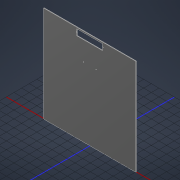
# Autodesk Inventor part: Panel Back
Saved by Autodesk Inventor 2022.2 (Build 262287010, 287A)
## iProperties
Created: 2022-03-16
Part Number: Panel Back
Material: Polycarbonat, klar
Document SubType Name: Modeling
Designer: sleib
Density: 1.2 g/cm^3
Appearance: Glatt - Schwarz
Author: sleib
Autodesk Inventor part; units mm, degrees
ref_plane "YZ Plane" through (0, 0, 0) normal (1, 0, 0) x (0, 1, 0)
ref_plane "XZ Plane" through (0, 0, 0) normal (0, 1, 0) x (-1, 0, 0)
ref_plane "XY Plane" through (0, 0, 0) normal (0, 0, 1) x (1, 0, 0)
sketch "Skizze1" plane through (0, 0, 0) normal (0, 0, 1) x (1, 0, 0)
  line L0 (-242, -252) -> (242, -252)
  line L1 (242, -252) -> (242, 252)
  line L2 (242, 252) -> (-242, 252)
  line L3 (-242, 252) -> (-242, -252)
  line L4 (-242, -252) -> (242, 252) construction
  line L5 (242, -252) -> (-242, 252) construction
  line L6 (-67.5, 245) -> (67.5, 245)
  line L7 (67.5, 213) -> (-67.5, 213)
  line L8 (0, 245) -> (0, 213) construction
  line L9 (69.1, 229) -> (-69.1, 229) construction
  line L10 (-69.1, 230.7) -> (-67.5, 230.7)
  line L11 (-69.1, 227.3) -> (-67.5, 227.3)
  line L12 (69.1, 230.7) -> (67.5, 230.7)
  line L13 (69.1, 227.3) -> (67.5, 227.3)
  line L14 (67.5, 245) -> (67.5, 230.7)
  line L15 (67.5, 227.3) -> (67.5, 213)
  arc A0 (69.1, 227.3) -> (69.1, 230.7) centre (69.1, 229) ccw
  arc A1 (-69.1, 230.7) -> (-69.1, 227.3) centre (-69.1, 229) ccw
  line L16 (-67.5, 230.7) -> (-67.5, 245)
  line L17 (-67.5, 213) -> (-67.5, 227.3)
  circle A2 centre (-33.4649, 111.0916) radius 1.7
  circle A3 centre (33.465, 111.0916) radius 1.7
  point P0 (0, 0)
  point P1 (0, 252)
  point P2 (0, 229)
  dimension "d0" = 484
  dimension "d1" = 504
  dimension "d6" = 135
  dimension "d7" = 32
  dimension "d8" = 138.2
  dimension "d10" = 3.4
  dimension "d11" = 117.9083
  dimension "d13" = 3.4
  dimension "d15" = 66.9299
  dimension "d16" = 7
  constraints: 36 end point, 13 perpendicular, 7 midpoint, 7 parallel, 4 centre point, 4 point on circle, 4 tangent, 2 equal radius, 2 horizontal, 2 symmetric about line, 1 collinear, 1 vertical alignment
  measures "d0" distance of L2.end L1.end
  measures "d1" distance of L2.end L0.start
  measures "d6" distance of L7.start L7.end
  measures "d7" distance between parallel lines of L7 L6
  measures "d8" distance of L9.start L9.end
  measures "d10" distance between parallel lines of L11 L10
  measures "d11" vertical distance of A3.centre L9.start
  measures "d13" diameter of A3
  measures "d15" distance of A3.centre A2.centre
  measures "d16" distance between parallel lines of L6 L2
extrude "Extrusion1" add sketch "Skizze1" along normal blind 3
